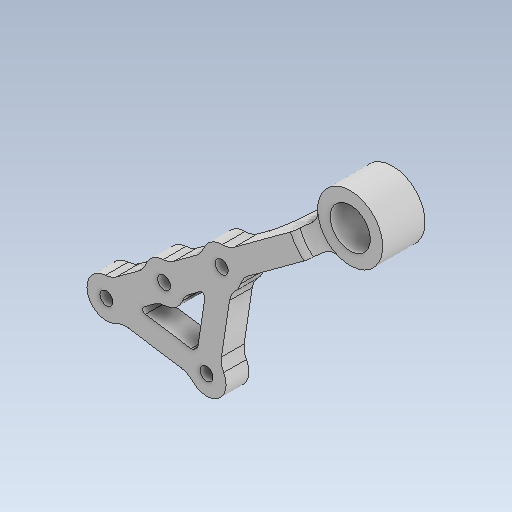
# Autodesk Inventor part: leg_link_4
Saved by Autodesk Inventor 2023 (Build 270158000, 158)
## iProperties
Created: 2020-12-12
Part Number: leg_link_4
Material: Generic
Document SubType Name: Modeling
Designer: Shuang Peng
Density: 1 g/cm^3
Appearance: Default
Author: Shuang Peng
Autodesk Inventor part; units mm, degrees
ref_plane "YZ Plane" through (0, 0, 0) normal (1, 0, 0) x (0, 1, 0)
ref_plane "XZ Plane" through (0, 0, 0) normal (0, 1, 0) x (-1, 0, 0)
ref_plane "XY Plane" through (0, 0, 0) normal (0, 0, 1) x (1, 0, 0)
sketch "Sketch1" plane through (0, 0, 0) normal (0, 0, 1) x (1, 0, 0)
  circle A0 centre (25.6771, -21.4815) radius 1.5 projected
  circle A1 centre (-16.2059, 21.4815) radius 1.5 projected
  line L0 (-25.0385, -0.8784) -> (-16.1909, 17.4815) projected
  arc A2 (-16.1909, 17.4815) -> (-19.3439, 19.0009) centre (-16.2059, 21.4815) ccw projected
  line L1 (-19.3439, 19.0009) -> (-29.5036, -2.0819) projected
  arc A3 (-29.5036, -2.0819) -> (-27.7754, -4.585) centre (-27.9271, -2.8416) ccw projected
  arc A4 (21.8157, -20.4378) -> (-27.7754, -4.585) centre (-22.7656, -74.4055) ccw projected
  arc A5 (21.8157, -20.4378) -> (24.1897, -17.7683) centre (25.6771, -21.4815) ccw projected
  arc A6 (24.1897, -17.7683) -> (-25.0385, -0.8784) centre (-21.5131, -70.7896) ccw projected
  circle A7 centre (25.6771, -21.4815) radius 5
  line L2 (-7.7058, -42.2888) -> (-12.4737, -40.7572) projected
  arc A8 (-12.4098, -39.7891) -> (-12.4737, -40.7572) centre (-12.3207, -40.2811) ccw projected
  line L3 (-12.4098, -39.7891) -> (-7.4821, -38.8967) projected
  arc A9 (-6.3198, -40.0581) -> (-7.4821, -38.8967) centre (-7.3039, -39.8807) ccw projected
  arc A10 (-6.3198, -40.0581) -> (-6.401, -41.2901) centre (-0.907, -41.0336) ccw projected
  arc A11 (-7.7058, -42.2888) -> (-6.401, -41.2901) centre (-7.3999, -41.3367) ccw projected
  line L4 (8.1067, -33.7799) -> (5.2533, -37.8953) projected
  arc A12 (3.6102, -37.896) -> (5.2533, -37.8953) centre (4.4315, -37.3255) ccw projected
  arc A13 (3.6102, -37.896) -> (2.7965, -36.9674) centre (-0.907, -41.0336) ccw projected
  arc A14 (3.0129, -35.3386) -> (2.7965, -36.9674) centre (3.4699, -36.2281) ccw projected
  line L5 (3.0129, -35.3386) -> (7.4674, -33.0502) projected
  arc A15 (8.1067, -33.7799) -> (7.4674, -33.0502) centre (7.6958, -33.495) ccw projected
  circle A16 centre (-10.7707, -36.1647) radius 1.6 projected
  circle A17 centre (3.962, -31.1699) radius 1.6 projected
  line L6 (0.0062, -25.0597) -> (-0.3734, -31.6998) projected
  arc A18 (-1.728, -33.4798) -> (-0.3734, -31.6998) centre (-2.3701, -31.5857) ccw projected
  line L7 (-1.728, -33.4798) -> (-4.8492, -34.538) projected
  arc A19 (-7.0069, -33.9488) -> (-4.8492, -34.538) centre (-5.4913, -32.6438) ccw projected
  line L8 (-7.0069, -33.9488) -> (-11.3465, -28.9086) projected
  arc A20 (-11.3465, -28.9086) -> (0.0062, -25.0597) centre (-0.907, -41.0336) ccw projected
  circle A21 centre (9.5106, -37.5018) radius 1.6 projected
  circle A22 centre (-11.3246, -44.5655) radius 1.6 projected
  circle A23 centre (2.6248, -51.4512) radius 1.6 projected
  line L9 (-10.8934, -48.4849) -> (-6.3871, -45.1225) projected
  arc A24 (-4.5079, -45.1909) -> (-6.3871, -45.1225) centre (-5.49, -46.3247) ccw projected
  arc A25 (-4.5079, -45.1909) -> (-2.0172, -46.4204) centre (-0.907, -41.0336) ccw projected
  arc A26 (-0.8201, -47.8705) -> (-2.0172, -46.4204) centre (-2.32, -47.8895) ccw projected
  line L10 (-0.8201, -47.8705) -> (-0.7487, -53.4925) projected
  arc A27 (-1.8159, -54.503) -> (-0.7487, -53.4925) centre (-1.7486, -53.5053) ccw projected
  arc A28 (-11.0465, -49.9466) -> (-1.8159, -54.503) centre (-0.907, -41.0336) ccw projected
  arc A29 (-10.8934, -48.4849) -> (-11.0465, -49.9466) centre (-10.2954, -49.2864) ccw projected
  arc A30 (8.006, -51.1731) -> (12.5624, -41.9425) centre (-0.907, -41.0336) ccw projected
  arc A31 (6.5443, -51.02) -> (8.006, -51.1731) centre (7.3457, -50.422) ccw projected
  line L11 (6.5443, -51.02) -> (3.1819, -46.5137) projected
  arc A32 (3.2503, -44.6346) -> (3.1819, -46.5137) centre (4.3841, -45.6166) ccw projected
  arc A33 (3.2503, -44.6346) -> (4.4798, -42.1438) centre (-0.907, -41.0336) ccw projected
  arc A34 (5.9299, -40.9467) -> (4.4798, -42.1438) centre (5.9489, -42.4466) ccw projected
  line L12 (5.9299, -40.9467) -> (11.5519, -40.8753) projected
  arc A35 (12.5624, -41.9425) -> (11.5519, -40.8753) centre (11.5646, -41.8752) ccw projected
  circle A36 centre (-0.907, -41.0336) radius 2.5 projected
  line L13 (25.6771, -21.4815) -> (-0.907, -41.0336)
  line L14 (-0.907, -41.0336) -> (7.9544, -34.5162)
  circle A37 centre (7.9544, -34.5162) radius 1
  line L15 (-0.907, -41.0336) -> (-9.7684, -47.551)
  circle A38 centre (-9.7684, -47.551) radius 1
  line L16 (7.9544, -34.5162) -> (-9.7684, -47.551) construction
  line L17 (6.7694, -32.9051) -> (-10.9533, -45.9398)
  line L18 (-8.5834, -49.1621) -> (9.1393, -36.1274)
  arc A39 (9.1393, -36.1274) -> (6.7694, -32.9051) centre (7.9544, -34.5162) ccw
  arc A40 (-10.9533, -45.9398) -> (-8.5834, -49.1621) centre (-9.7684, -47.551) ccw
  line L19 (25.6771, -21.4815) -> (7.9544, -34.5162) construction
  line L20 (24.6402, -20.0717) -> (6.9175, -33.1065)
  line L21 (8.9912, -35.926) -> (26.714, -22.8912)
  arc A41 (26.714, -22.8912) -> (24.6402, -20.0717) centre (25.6771, -21.4815) ccw
  arc A42 (6.9175, -33.1065) -> (8.9912, -35.926) centre (7.9544, -34.5162) ccw
  line L22 (7.9544, -34.5162) -> (9.1393, -36.1274)
  line L23 (7.9544, -34.5162) -> (6.7694, -32.9051)
  point P0 (0, 0)
  point P1 (16.8157, -27.9989)
  point P2 (22.9408, -25.6663)
  point P3 (20.8671, -22.8468)
  dimension "d0" = 10
  dimension "d1" = 11
  dimension "d2" = 2
  dimension "d3" = 11
  dimension "d4" = 2
  dimension "d5" = 4
  dimension "d6" = 3.5
  constraints: 26 end point, 8 point on circle, 8 tangent, 7 centre point, 4 collinear, 3 coincident, 2 midpoint, 2 parallel, 2 perpendicular
  measures "d0" diameter of A7
  measures "d1" distance of L13.end L14.end
  measures "d2" diameter of A37
  measures "d3" distance of L13.end L15.end
  measures "d4" diameter of A38
  measures "d5" diameter of A40
  measures "d6" diameter of A42
extrude "Extrusion1" add sketch "Sketch1" along normal blind 7 contours A0 | A7 L21 A5 A6 | A6 A5 L21 A41 L20 A4 A7 | A4 A5 L20 A7 | L21 A7 L13 A5 | A5 L20 A41 L21 | L21 A20 L13 A7 | L20 A5 L13 A7 | A7 L13 A20 L20 | L21 A39 L13 A20 | A20 L13 A39 L20 | L21 L22 A37 L13 A39 | A39 L13 A37 A15 L5 L23 L20 | L22 A21 L18 A36 L13 A13 A12 L4 A42 | A42 L4 A37 L22 | L23 A42 L5 L17 | L23 L5 A42 | L22 L18 A21 | A42 L13 A37 L4 | L4 A12 A13 L13 A42 | L5 A42 L13 A13 A14 L17 | L5 L23 A37 L13 A42 | L5 A15 A37 L23 | A14 A13 L13 A36 L17 | L18 A36 L15 L13 | A36 L13 L15 L17 | L18 A25 A24 L9 A38 L15 A36 | A36 L15 A38 L9 A29 A40 A22 L17 | L18 A40 A29 L9 A38 A24 A25 | A22 A40 L17 picked at (-10.251, -45.4933)
sketch "Sketch2" plane through (0, 0, 0) normal (0, 0, -1) x (-1, 0, 0)
  line L0 (-6.9175, -33.1065) -> (-6.7694, -32.9051) projected
  line L1 (-20.8671, -22.8468) -> (-6.9175, -33.1065) projected
  arc A0 (-20.8671, -22.8468) -> (-22.9408, -25.6663) centre (-25.6771, -21.4815) ccw projected
  line L2 (-8.9912, -35.926) -> (-22.9408, -25.6663) projected
  line L3 (-9.1393, -36.1274) -> (-8.9912, -35.926) projected
  line L4 (8.5834, -49.1621) -> (-9.1393, -36.1274) projected
  arc A1 (8.5834, -49.1621) -> (10.9533, -45.9398) centre (9.7684, -47.551) ccw projected
  line L5 (-6.7694, -32.9051) -> (10.9533, -45.9398) projected
  circle A2 centre (-7.9544, -34.5162) radius 1 projected
  circle A3 centre (9.7684, -47.551) radius 1 projected
  line L6 (-7.9544, -34.5162) -> (-16.0102, -28.5913)
  line L7 (-7.9544, -34.5162) -> (-25.6771, -21.4815)
  line L8 (-16.0102, -28.5913) -> (-14.9733, -27.1816)
  line L9 (-16.0102, -28.5913) -> (-17.047, -30.0011)
  line L10 (-8.9912, -35.926) -> (-22.9408, -25.6663) projected
  point P0 (0, 0)
  dimension "d9" = 10
  constraints: 8 end point, 2 perpendicular, 2 point on line, 1 collinear
  measures "d9" distance of L6.start L6.end
ref_plane "Work Plane1" through (-30.8639, -71.7439, 5) normal (0, 0, 1) x (0.9470532, 0.3210766, 0)
extrude "Extrusion2" cut sketch "Sketch2" against normal up to surface (5 mm away) contours L0 L5 A1 L4 L3 L2 L9 L8 L1
thicken "Thicken1" operation add thickness 1.5 both sides no extend neighbours yes toward (0, 0, 1) faces at (17.5036, -27.4554, 7)
sketch "Sketch3" plane through (25.6771, -21.4815, 8.5) normal (0, 0, 1) x (0.8055786, 0.5924889, 0)
  line L0 (-22, 1.75) -> (-22, 2) projected
  line L1 (-22, 2) -> (-44, 2) projected
  arc A0 (-44, 2) -> (-44, -2) centre (-44, 0) ccw projected
  line L2 (-44, -2) -> (-22, -2) projected
  line L3 (-22, -2) -> (-22, -1.75) projected
  line L4 (-22, -1.75) -> (-4.6837, -1.75) projected
  arc A1 (-4.6837, -1.75) -> (-4.6837, 1.75) centre (0, 0) ccw projected
  line L5 (-4.6837, 1.75) -> (-22, 1.75) projected
  circle A2 centre (-22, 0) radius 1 projected
  circle A3 centre (-44, 0) radius 1 projected
  circle A4 centre (-44, 0) radius 3
  circle A5 centre (-22, 0) radius 1 projected
  circle A6 centre (-22, 0) radius 3
  point P0 (-7.9574, 32.5184)
  point P1 (-19.5633, 1.75)
  point P2 (-24.2361, 2)
  point P3 (-24.2361, -2)
  point P4 (-19.5633, -1.75)
  point P5 (-41.7639, 2)
  point P6 (-41.7639, -2)
  dimension "d14" = 6
  dimension "d15" = 6
  constraints: 2 centre point, 2 coincident
  measures "d14" diameter of A4
  measures "d15" diameter of A6
extrude "Extrusion3" add sketch "Sketch3" against normal up to surface (3.5 mm away) contours L0 L1 A6 L5 | L1 A0 L2 A4 | L2 L3 L4 A6 picked at (-42.6901, 2.1587)
sketch "Sketch4" plane through (25.6771, -21.4815, 8.5) normal (0, 0, 1) x (0.8055786, 0.5924889, 0)
  arc A0 (-19.5633, 1.75) -> (-24.2361, 2) centre (-22, 0) ccw projected
  line L0 (-24.2361, 2) -> (-41.7639, 2) projected
  arc A1 (-41.7639, 2) -> (-41.7639, -2) centre (-44, 0) ccw projected
  line L1 (-41.7639, -2) -> (-24.2361, -2) projected
  arc A2 (-24.2361, -2) -> (-19.5633, -1.75) centre (-22, 0) ccw projected
  line L2 (-19.5633, -1.75) -> (-4.6837, -1.75) projected
  arc A3 (-4.6837, -1.75) -> (-4.6837, 1.75) centre (0, 0) ccw projected
  line L3 (-4.6837, 1.75) -> (-19.5633, 1.75) projected
  circle A4 centre (-22, 0) radius 1 projected
  circle A5 centre (-44, 0) radius 1 projected
  circle A6 centre (0, 0) radius 3.075
  point P0 (-7.9574, 32.5184)
  dimension "d18" = 6.15
  constraints: 1 centre point, 1 coincident
  measures "d18" diameter of A6
extrude "Extrusion4" cut sketch "Sketch4" against normal blind 9 contours A6
sketch "Sketch5" plane through (25.6771, -21.4815, 8.5) normal (0, 0, 1) x (0.8055786, 0.5924889, 0)
  circle A0 centre (0, 0) radius 3.075 projected
  arc A1 (-19.5633, 1.75) -> (-24.2361, 2) centre (-22, 0) ccw projected
  line L0 (-24.2361, 2) -> (-41.7639, 2) projected
  arc A2 (-41.7639, 2) -> (-41.7639, -2) centre (-44, 0) ccw projected
  line L1 (-41.7639, -2) -> (-24.2361, -2) projected
  arc A3 (-24.2361, -2) -> (-19.5633, -1.75) centre (-22, 0) ccw projected
  line L2 (-19.5633, -1.75) -> (-4.6837, -1.75) projected
  arc A4 (-4.6837, -1.75) -> (-4.6837, 1.75) centre (0, 0) ccw projected
  line L3 (-4.6837, 1.75) -> (-19.5633, 1.75) projected
  circle A5 centre (-22, 0) radius 1 projected
  circle A6 centre (-44, 0) radius 1 projected
  circle A7 centre (-22, 0) radius 1 projected
  circle A8 centre (-44, 0) radius 1 projected
  line L4 (-22, 0) -> (-44, 0)
  circle A9 centre (-33, 0) radius 1
  point P0 (-7.9574, 32.5184)
  dimension "d21" = 2
  constraints: 2 end point, 1 centre point, 1 horizontal, 1 midpoint
  measures "d21" diameter of A9
extrude "Extrusion5" cut sketch "Sketch5" against normal blind 9 contours A9 L4 | L4 A9
sketch "Sketch6" plane through (25.6771, -21.4815, 8.5) normal (0, 0, 1) x (0.8055786, 0.5924889, 0)
  circle A0 centre (-33, 0) radius 1 projected
  circle A1 centre (0, 0) radius 3.075 projected
  arc A2 (-19.5633, 1.75) -> (-24.2361, 2) centre (-22, 0) ccw projected
  line L0 (-24.2361, 2) -> (-41.7639, 2) projected
  arc A3 (-41.7639, 2) -> (-41.7639, -2) centre (-44, 0) ccw projected
  line L1 (-41.7639, -2) -> (-24.2361, -2) projected
  arc A4 (-24.2361, -2) -> (-19.5633, -1.75) centre (-22, 0) ccw projected
  line L2 (-19.5633, -1.75) -> (-4.6837, -1.75) projected
  arc A5 (-4.6837, -1.75) -> (-4.6837, 1.75) centre (0, 0) ccw projected
  line L3 (-4.6837, 1.75) -> (-19.5633, 1.75) projected
  circle A6 centre (-22, 0) radius 1 projected
  circle A7 centre (-44, 0) radius 1 projected
  circle A8 centre (0, 0) radius 7
  point P0 (-7.9574, 32.5184)
  dimension "d24" = 14
  constraints: 1 centre point, 1 coincident
  measures "d24" diameter of A8
extrude "Extrusion6" cut sketch "Sketch6" against normal blind 2 contours A8 L2 A5 L3 | L3 A5 L2 A8
fillet "Fillet1" radius 4 1 edges at (16.0102, -28.5913, 5)
fillet "Fillet2" radius 2 1 edges at (16.0102, -28.5913, 0)
fillet "Fillet3" radius 2 2 edges at (22.9408, -25.6663, 3.25) (20.8671, -22.8468, 3.25)
fillet "Fillet4" radius 2 1 edges at (20.038, -25.6289, 6.5)
fillet "Fillet5" radius 1 4 edges at (19.1803, -24.0874, 8.5) (20.038, -25.6289, 8.4999) (21.254, -26.907, 8.5) (20.038, -25.6289, 8.5)
sketch "Sketch7" plane through (-9.7684, -47.551, 8.5) normal (0, 0, 1) x (0.8055786, 0.5924889, 0)
  arc A0 (36.3697, 1.75) -> (36.3697, -1.75) centre (44, 0) ccw projected
  line L0 (36.3697, 1.75) -> (24.4367, 1.75) projected
  arc A1 (24.4367, 1.75) -> (19.7639, 2) centre (22, 0) ccw projected
  line L1 (19.7639, 2) -> (2.2361, 2) projected
  arc A2 (2.2361, 2) -> (2.2361, -2) centre (0, 0) ccw projected
  line L2 (2.2361, -2) -> (19.7639, -2) projected
  arc A3 (19.7639, -2) -> (24.4367, -1.75) centre (22, 0) ccw projected
  line L3 (24.4367, -1.75) -> (36.3697, -1.75) projected
  circle A4 centre (11, 0) radius 1 projected
  circle A5 centre (22, 0) radius 1 projected
  circle A6 centre (0, 0) radius 1 projected
  circle A7 centre (11, 0) radius 1 projected
  circle A8 centre (11, 0) radius 3
  point P0 (36.0426, 32.5184)
  point P1 (8.7639, 2)
  point P2 (13.2361, 2)
  point P3 (13.2361, -2)
  point P4 (8.7639, -2)
  dimension "d35" = 6
  constraints: 1 centre point, 1 coincident
  measures "d35" diameter of A8
extrude "Extrusion7" add sketch "Sketch7" against normal blind 3.5 contours L1 A8 | A8 L2
sketch "Sketch8" plane through (-9.7684, -47.551, 8.5) normal (0, 0, 1) x (0.8055786, 0.5924889, 0)
  arc A0 (36.3697, 1.75) -> (36.3697, -1.75) centre (44, 0) ccw projected
  line L0 (36.3697, 1.75) -> (24.4367, 1.75) projected
  arc A1 (24.4367, 1.75) -> (19.7639, 2) centre (22, 0) ccw projected
  line L1 (19.7639, 2) -> (13.2361, 2) projected
  arc A2 (13.2361, 2) -> (8.7639, 2) centre (11, 0) ccw projected
  line L2 (8.7639, 2) -> (2.2361, 2) projected
  arc A3 (2.2361, 2) -> (2.2361, -2) centre (0, 0) ccw projected
  line L3 (2.2361, -2) -> (8.7639, -2) projected
  arc A4 (8.7639, -2) -> (13.2361, -2) centre (11, 0) ccw projected
  line L4 (13.2361, -2) -> (19.7639, -2) projected
  arc A5 (19.7639, -2) -> (24.4367, -1.75) centre (22, 0) ccw projected
  line L5 (24.4367, -1.75) -> (36.3697, -1.75) projected
  circle A6 centre (11, 0) radius 1 projected
  circle A7 centre (22, 0) radius 1 projected
  circle A8 centre (0, 0) radius 1 projected
  line L6 (11, 0) -> (11, -11)
  circle A9 centre (11, -11) radius 1
  circle A10 centre (11, -11) radius 1.75
  line L7 (22, 0) -> (11, -11) construction
  line L8 (20.7626, 1.2374) -> (9.7626, -9.7626)
  line L9 (12.2374, -12.2374) -> (23.2374, -1.2374)
  arc A11 (23.2374, -1.2374) -> (20.7626, 1.2374) centre (22, 0) ccw
  arc A12 (9.7626, -9.7626) -> (12.2374, -12.2374) centre (11, -11) ccw
  line L10 (11, -11) -> (0, 0) construction
  line L11 (13.1213, -8.8787) -> (2.1213, 2.1213)
  line L12 (-2.1213, -2.1213) -> (8.8787, -13.1213)
  arc A13 (8.8787, -13.1213) -> (13.1213, -8.8787) centre (11, -11) ccw
  arc A14 (2.1213, 2.1213) -> (-2.1213, -2.1213) centre (0, 0) ccw
  circle A15 centre (0, 0) radius 1 projected
  line L13 (11, -11) -> (0, 0) construction
  line L14 (12.2374, -9.7626) -> (1.2374, 1.2374)
  line L15 (-1.2374, -1.2374) -> (9.7626, -12.2374)
  arc A16 (9.7626, -12.2374) -> (12.2374, -9.7626) centre (11, -11) ccw
  arc A17 (1.2374, 1.2374) -> (-1.2374, -1.2374) centre (0, 0) ccw
  circle A18 centre (11, -11) radius 3
  point P0 (36.0426, 32.5184)
  point P1 (16.5, -5.5)
  point P2 (5.5, -5.5)
  point P3 (5.5, -5.5)
  point P4 (10.5144, -8.0396)
  point P5 (4.4749, -2)
  point P6 (0.4856, -2.9604)
  point P7 (8.0396, -10.5144)
  point P8 (8.8787, -13.1213)
  point P9 (13.9604, -10.5144)
  point P10 (21.5144, -2.9604)
  point P11 (17.5251, -2)
  point P12 (11.4856, -8.0396)
  dimension "d38" = 11
  dimension "d39" = 2
  dimension "d40" = 3.5
  dimension "d42" = 6
  dimension "d43" = 3.5
  dimension "d44" = 6
  constraints: 26 end point, 12 point on circle, 12 tangent, 9 centre point, 3 coincident, 3 midpoint, 3 parallel, 2 concentric, 1 vertical
  measures "d38" distance of L6.start L6.end
  measures "d39" diameter of A9
  measures "d40" diameter of A10
  measures "d42" diameter of A14
  measures "d43" diameter of A17
  measures "d44" diameter of A18
extrude "Extrusion8" add sketch "Sketch8" against normal blind 3.5 contours L9 A13 L11 L8 L4 A5 | A13 A18 L15 A10 L9 | L9 A10 L14 L8 A18 A13 | A10 | A18 L8 L11 | L15 A18 L14 L8 A10 | L8 L6 A18 | L8 L6 A10 | L15 A3 L3 L14 A18 | A10 L6 L14 | L14 A18 L6
fillet "Fillet6" radius 3 12 edges at (-9.152, -44.615, 6.75) (-3.8933, -40.7473, 6.75) (-0.2906, -38.0976, 6.75) (4.9681, -34.2299, 6.75) (8.8805, -31.6628, 6.75) (10.9542, -34.4823, 6.75) (9.3172, -37.1888, 6.75) (7.7076, -47.7498, 6.75) (2.9378, -51.2578, 6.75) (-7.6232, -49.6482, 6.75) (-1.5233, -43.9696, 6.75) (2.0793, -41.3199, 6.75)
fillet "Fillet7" radius 0.5 4 edges at (-4.9785, -46.5108, 6.75) (3.4652, -47.7978, 6.75) (4.2475, -47.2224, 6.75) (5.5345, -38.7787, 6.75)
body "Solid1"
